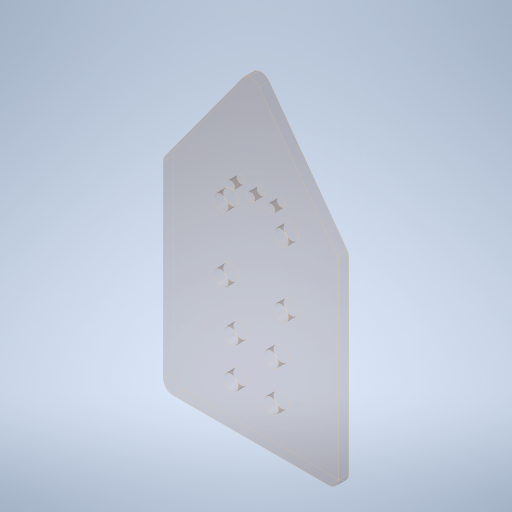
# Autodesk Inventor part: CL7-017
Saved by Autodesk Inventor 2023.4 (Build 274418000, 418)
## iProperties
Created: 2025-03-19
Part Number: CL7-017
Material: Polycarbonate, Smoke
Document SubType Name: Modeling
Designer: slick
Density: 1.2 g/cm^3
Appearance: Polycarbonate - Smoked
Author: slick
Autodesk Inventor part; units mm, degrees
ref_plane "YZ Plane" through (0, 0, 0) normal (1, 0, 0) x (0, 1, 0)
ref_plane "XZ Plane" through (0, 0, 0) normal (0, 1, 0) x (-1, 0, 0)
ref_plane "XY Plane" through (0, 0, 0) normal (0, 0, 1) x (1, 0, 0)
sketch "Sketch1" plane through (0, 0, 0) normal (0, 0, 1) x (1, 0, 0)
  line L0 (55.5625, 0) -> (-55.5625, 0)
  line L1 (-55.5625, 0) -> (0, 76.2)
  line L2 (0, 76.2) -> (55.5625, 0)
  line L3 (-55.5625, 0) -> (55.5625, 0)
  line L4 (55.5625, 0) -> (55.5625, -127)
  line L5 (55.5625, -127) -> (-55.5625, -127)
  line L6 (-55.5625, -127) -> (-55.5625, 0)
  point P0 (0, 0)
  point P1 (0, 0)
  dimension "d0" = 111.125
  dimension "d1" = 76.2
  dimension "d14" = 127
  constraints: 15 end point, 2 coincident, 2 horizontal, 2 parallel, 1 equal length, 1 midpoint, 1 perpendicular, 1 vertical alignment
  measures "d0" distance of L0.start L0.end
  measures "d1" distance from line of L0 L1.end
  measures "d14" distance between parallel lines of L0 L5
extrude "Extrusion1" add sketch "Sketch1" along normal blind 6.35
sketch "Sketch2" plane through (0, 0, 6.35) normal (0, 0, 1) x (1, 0, 0)
  line L0 (-12.7, 6.35) -> (12.7, 6.35) construction
  line L1 (-55.5625, -127) -> (55.5625, -127) construction
  point P0 (0, 6.35)
  point P1 (0, 6.35)
  point P2 (0, 76.2)
  dimension "d6" = 25.4
  dimension "d15" = 133.35
  constraints: 2 end point, 2 horizontal alignment, 1 coincident, 1 horizontal, 1 midpoint, 1 vertical alignment
  measures "d6" distance of L0.start L0.end
  measures "d15" distance from line of L0.start L1
hole "Hole1" at (-12.7, 6.35, 6.35) at (0, 6.35, 6.35) at (12.7, 6.35, 6.35) direction (0, 0, -1) diameter 5.1054 end through all start extended yes clearance for "Flat Head Machine Screw (82)" size "#10" standard "Ansi Unified Screw Threads"
fillet "Fillet2" radius 6.35 5 edges at (-55.5625, 0, 3.175) (55.5625, 0, 3.175) (0, 76.2, 3.175) (-55.5625, -127, 3.175) (55.5625, -127, 3.175)
sketch "Sketch3" plane through (0, 0, 6.35) normal (0, 0, 1) x (1, 0, 0)
  arc A0 (49.2125, -127) -> (55.5625, -120.65) centre (49.2125, -120.65) ccw construction
  line L0 (55.5625, -120.65) -> (55.5625, -2.0693) construction
  arc A1 (55.5625, -2.0693) -> (54.3433, 1.672) centre (49.2125, -2.0693) ccw construction
  line L1 (54.3433, 1.672) -> (5.1308, 69.1634) construction
  arc A2 (5.1308, 69.1634) -> (-5.1308, 69.1634) centre (0, 65.4222) ccw construction
  line L2 (-5.1308, 69.1634) -> (-54.3433, 1.672) construction
  arc A3 (-54.3433, 1.672) -> (-55.5625, -2.0693) centre (-49.2125, -2.0693) ccw construction
  line L3 (-55.5625, -2.0693) -> (-55.5625, -120.65) construction
  arc A4 (-55.5625, -120.65) -> (-49.2125, -127) centre (-49.2125, -120.65) ccw construction
  line L4 (-49.2125, -127) -> (49.2125, -127) construction
  circle A5 centre (0, 6.35) radius 2.5527 construction
  circle A6 centre (-12.7, 6.35) radius 2.5527 construction
  circle A7 centre (12.7, 6.35) radius 2.5527 construction
  line L5 (0, 31.75) -> (-30.7945, 0.9555) construction
  line L6 (0, 31.75) -> (30.7945, 0.9555) construction
  point P0 (0, 0)
  dimension "d17" = 25.4
  constraints: 4 end point, 2 perpendicular, 1 horizontal alignment, 1 vertical alignment
  measures "d17" distance of A5.centre L5.start
sketch "Sketch4" plane through (0, 0, 6.35) normal (0, 0, 1) x (1, 0, 0)
  arc A0 (49.2125, -127) -> (55.5625, -120.65) centre (49.2125, -120.65) ccw construction
  line L0 (55.5625, -120.65) -> (55.5625, -2.0693) construction
  arc A1 (55.5625, -2.0693) -> (54.3433, 1.672) centre (49.2125, -2.0693) ccw construction
  line L1 (54.3433, 1.672) -> (5.1308, 69.1634) construction
  arc A2 (5.1308, 69.1634) -> (-5.1308, 69.1634) centre (0, 65.4222) ccw construction
  line L2 (-5.1308, 69.1634) -> (-54.3433, 1.672) construction
  arc A3 (-54.3433, 1.672) -> (-55.5625, -2.0693) centre (-49.2125, -2.0693) ccw construction
  line L3 (-55.5625, -2.0693) -> (-55.5625, -120.65) construction
  arc A4 (-55.5625, -120.65) -> (-49.2125, -127) centre (-49.2125, -120.65) ccw construction
  line L4 (-49.2125, -127) -> (49.2125, -127) construction
  circle A5 centre (0, 6.35) radius 2.5527 construction
  circle A6 centre (-12.7, 6.35) radius 2.5527 construction
  circle A7 centre (12.7, 6.35) radius 2.5527 construction
  point P0 (0, 0)
  point P1 (-12.7, -101.6)
  point P2 (-12.7, -76.2)
  point P3 (-19.05, -47.625)
  point P4 (-19.05, -6.35)
  dimension "d24" = 12.7
  dimension "d25" = 19.05
  dimension "d26" = 53.975
  dimension "d27" = 19.05
  dimension "d28" = 12.7
  dimension "d29" = 82.55
  dimension "d30" = 107.95
  constraints: 1 vertical alignment
  measures "d24" vertical distance of A5.centre point (-19.05, -6.35)
  measures "d25" horizontal distance of A5.centre point (-19.05, -6.35)
  measures "d26" vertical distance of point (-19.05, -47.625) A5.centre
  measures "d27" horizontal distance of A5.centre point (-19.05, -47.625)
  measures "d28" horizontal distance of point (-12.7, -76.2) A5.centre
  measures "d29" vertical distance of point (-12.7, -76.2) A5.centre
  measures "d30" vertical distance of A7.centre point (-12.7, -101.6)
hole "Hole2" at (-12.7, -101.6, 6.35) at (-12.7, -76.2, 6.35) at (-19.05, -47.625, 6.35) at (-19.05, -6.35, 6.35) direction (0, 0, -1) diameter 9.525 end through all
mirror "Mirror1" about plane through (0, 0, 0) normal (1, 0, 0) of "Hole2"
body "Solid1"
